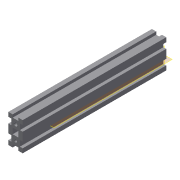
# Autodesk Inventor part: Neje_Base_Rod_20mm
Saved by Autodesk Inventor 2019.4 (Build 234330000, 330)
## iProperties
Created: 2021-06-27
Part Number: Neje_Base_Rod_20mm
Material: Generic
Document SubType Name: Modeling
Designer: diederichbenedict
Density: 1 g/cm^3
Appearance: Default
Mass: 102.36 g
Surface Area: 466.785 cm^2
Volume: 102.36 cm^3
Author: diederichbenedict
Autodesk Inventor part; units mm, degrees
ref_plane "YZ Plane" through (0, 0, 0) normal (1, 0, 0) x (0, 1, 0)
ref_plane "XZ Plane" through (0, 0, 0) normal (0, 1, 0) x (-1, 0, 0)
ref_plane "XY Plane" through (0, 0, 0) normal (0, 0, 1) x (1, 0, 0)
sketch "Sketch1" plane through (0, 0, 0) normal (0, 0, 1) x (1, 0, 0)
  line L0 (10, -10) -> (-10, 10) construction
  line L1 (-10, -10) -> (10, 10) construction
  line L2 (-4, 6) -> (4, 6)
  line L3 (4, 6) -> (4, 14)
  line L4 (4, 14) -> (-4, 14)
  line L5 (-4, 14) -> (-4, 6)
  line L6 (-4, 6) -> (4, 14) construction
  line L7 (4, 6) -> (-4, 14) construction
  line L8 (14, -4) -> (6, -4)
  line L9 (6, -4) -> (6, 4)
  line L10 (6, 4) -> (14, 4)
  line L11 (14, 4) -> (14, -4)
  line L12 (14, -4) -> (6, 4) construction
  line L13 (6, -4) -> (14, 4) construction
  line L14 (-4, -6) -> (4, -6)
  line L15 (4, -6) -> (4, -14)
  line L16 (4, -14) -> (-4, -14)
  line L17 (-4, -14) -> (-4, -6)
  line L18 (-4, -6) -> (4, -14) construction
  line L19 (4, -6) -> (-4, -14) construction
  line L20 (-14, 4) -> (-6, 4)
  line L21 (-6, 4) -> (-6, -4)
  line L22 (-6, -4) -> (-14, -4)
  line L23 (-14, -4) -> (-14, 4)
  line L24 (-14, 4) -> (-6, -4) construction
  line L25 (-6, 4) -> (-14, -4) construction
  line L26 (-10, -10) -> (-10, 0)
  line L27 (-10, 4) -> (-10, 10)
  line L28 (-10, 10) -> (0, 10)
  line L29 (4, 10) -> (10, 10)
  line L30 (10, 10) -> (10, 4)
  line L31 (10, 0) -> (10, -10)
  line L32 (10, -10) -> (4, -10)
  line L33 (0, -10) -> (-10, -10)
  point P0 (0, 0)
  point P1 (-4, 10)
  point P2 (10, -4)
  point P3 (-4, -10)
  point P4 (-10, -4)
  dimension "d0" = 20
  dimension "d1" = 20
  dimension "d2" = 8
  dimension "d3" = 8
  dimension "d4" = 8
  dimension "d5" = 8
  dimension "d6" = 8
  dimension "d7" = 8
  dimension "d8" = 8
  dimension "d9" = 8
  constraints: 68 end point, 18 midpoint, 16 parallel, 8 perpendicular, 6 horizontal, 4 coincident, 4 point on line
  measures "d0" distance of L0.end L1.end
  measures "d1" distance of L1.start L0.end
  measures "d2" distance of L4.end L3.end
  measures "d3" distance of L3.end L2.end
  measures "d4" distance of L9.end L10.end
  measures "d5" distance of L8.end L9.end
  measures "d6" distance of L15.end L16.end
  measures "d7" distance of L14.end L15.end
  measures "d8" distance of L21.end L22.end
  measures "d9" distance of L20.end L21.end
extrude "Extrusion1" add sketch "Sketch1" along normal blind 200 contours L2 L3 L29 L30 L10 L9 L8 L31 L32 L15 L14 L17 L33 L26 L22 L21 L20 L27 L28 L5
ref_plane "Work Plane1" through (4, 0, 0) normal (0, 1, 0) x (1, 0, 0)
ref_plane "Work Plane2" through (0, -10, 0) normal (1, 0, 0) x (0, 0, -1)
mirror "Mirror1" about plane through (10, 10, 0) normal (0, 1, 0) of "Extrusion1"
sketch "Sketch2" plane through (0, 0, 200) normal (0, 0, 1) x (1, 0, 0)
  line L0 (-10, 4) -> (-10, 16) projected
  line L1 (-10, 4) -> (-6, 4) projected
  line L2 (-6, 4) -> (-6, -4) projected
  line L3 (-6, -4) -> (-10, -4) projected
  line L4 (-10, -4) -> (-10, -10) projected
  line L5 (-10, -10) -> (-4, -10) projected
  line L6 (-4, -10) -> (-4, -6) projected
  line L7 (-4, -6) -> (4, -6) projected
  line L8 (4, -6) -> (4, -10) projected
  line L9 (4, -10) -> (10, -10) projected
  line L10 (10, -10) -> (10, -4) projected
  line L11 (10, -4) -> (6, -4) projected
  line L12 (6, -4) -> (6, 4) projected
  line L13 (6, 4) -> (10, 4) projected
  line L14 (10, 4) -> (10, 16) projected
  line L15 (6, 16) -> (10, 16) projected
  line L16 (6, 24) -> (6, 16) projected
  line L17 (10, 24) -> (6, 24) projected
  line L18 (10, 30) -> (10, 24) projected
  line L19 (4, 30) -> (10, 30) projected
  line L20 (4, 26) -> (4, 30) projected
  line L21 (-4, 26) -> (4, 26) projected
  line L22 (-4, 30) -> (-4, 26) projected
  line L23 (-10, 30) -> (-4, 30) projected
  line L24 (-10, 24) -> (-10, 30) projected
  line L25 (-6, 24) -> (-10, 24) projected
  line L26 (-6, 16) -> (-6, 24) projected
  line L27 (-10, 16) -> (-6, 16) projected
  line L28 (-4, 6) -> (-4, 14) projected
  line L29 (4, 14) -> (-4, 14) projected
  line L30 (4, 6) -> (4, 14) projected
  line L31 (4, 6) -> (-4, 6) projected
  circle A0 centre (0, 20) radius 2.5
  circle A1 centre (0, 0) radius 2
  point P0 (0, 0)
  dimension "d12" = 5
  dimension "d13" = 4
  dimension "d14" = 20
  dimension "d15" = 10
  constraints: 2 centre point
  measures "d12" diameter of A0
  measures "d13" diameter of A1
  measures "d14" distance of A1.centre A0.centre
  measures "d15" distance from line of A0.centre L19
extrude "Extrusion2" cut sketch "Sketch2" against normal through all contours A0 | A1
ref_plane "Work Plane3" through (0, 4, 200) normal (1, 0, 0) x (0, 0, -1)
body "Solid1"
